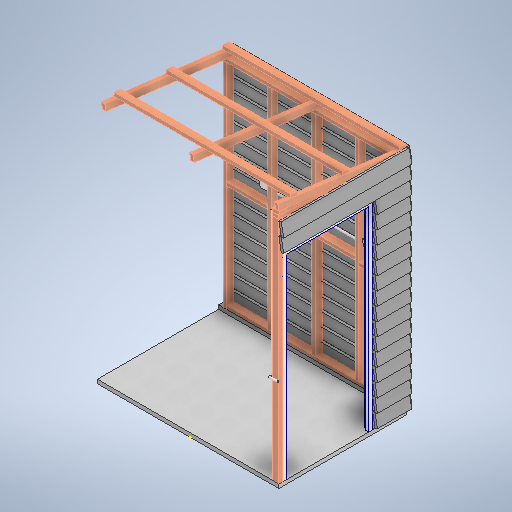
# Autodesk Inventor part: MaximaShed
Saved by Autodesk Inventor 2025 (Build 290162010, 162A)
## iProperties
Created: 2024-08-20
Part Number: MaximaShed
Material: Generic
Document SubType Name: Modeling
Designer: max_d
Density: 1 g/cm^3
Appearance: Default
Author: max_d
Autodesk Inventor part; units mm, degrees
ref_plane "YZ Plane" through (0, 0, 0) normal (1, 0, 0) x (0, 1, 0)
ref_plane "XZ Plane" through (0, 0, 0) normal (0, 1, 0) x (-1, 0, 0)
ref_plane "XY Plane" through (0, 0, 0) normal (0, 0, 1) x (1, 0, 0)
sketch "Sketch1" plane through (0, 0, 0) normal (0, 1, 0) x (-1, 0, 0)
  line L0 (0, 0) -> (-1850, 0)
  line L1 (-1850, 0) -> (-1850, -1235)
  line L2 (-1850, -1235) -> (0, -1235)
  line L3 (0, -1235) -> (0, 0)
  line L4 (0, -1235) -> (-1850, -1235)
  line L5 (-1850, -1235) -> (-1850, -1305)
  line L6 (-1850, -1305) -> (0, -1305)
  line L7 (0, -1305) -> (0, -1235)
  line L8 (-1850, -1235) -> (-1780, -1235)
  line L9 (-1780, -1235) -> (-1780, -975)
  line L10 (-1780, -975) -> (-1850, -975)
  line L11 (-1850, -975) -> (-1850, -1235)
  line L12 (-1780, -1105) -> (-1850, -1105) construction
  line L13 (-1744.6984, -1305) -> (-1744.6984, -1235) construction
  dimension "d0" = 1850
  dimension "d1" = 1235
  dimension "d5" = 70
  dimension "d19" = 260
  constraints: 28 end point, 6 parallel, 5 perpendicular, 3 horizontal, 2 midpoint, 2 point on line, 1 collinear
  measures "d0" distance of L2.end L1.end
  measures "d1" distance of L1.end L0.end
  measures "d5" distance of L5.end L4.end
  measures "d19" distance of L8.end L9.end
extrude "Extrusion1" add sketch "Sketch1" along normal blind 40 contours L3 L2 L9 L10 L1 L0 | L10 L9 L2 L1
extrude "Extrusion2" add sketch "Sketch1" along normal blind 80 contours L7 L6 L5 L2 | L10 L9 L2 L1
sketch "Sketch2" plane through (0, 80, 0) normal (0, 1, 0) x (1, 0, 0)
  line L0 (1850, 1305) -> (0, 1305) projected
  line L1 (0, 1235) -> (1780, 1235) projected
  line L2 (85, 1305) -> (85, 1235)
  line L3 (85, 1235) -> (50, 1235)
  line L4 (50, 1235) -> (50, 1305)
  line L5 (500, 1305) -> (535, 1305)
  line L6 (535, 1305) -> (535, 1235)
  line L7 (535, 1235) -> (500, 1235)
  line L8 (500, 1235) -> (500, 1305)
  line L9 (950, 1305) -> (985, 1305)
  line L10 (985, 1305) -> (985, 1235)
  line L11 (985, 1235) -> (950, 1235)
  line L12 (950, 1235) -> (950, 1305)
  line L13 (1395, 1305) -> (1430, 1305)
  line L14 (1430, 1305) -> (1430, 1235)
  line L15 (1430, 1235) -> (1395, 1235)
  line L16 (1395, 1235) -> (1395, 1305)
  line L17 (1850, 0) -> (1850, 1305) projected
  line L18 (1850, 1305) -> (1815, 1305)
  line L19 (1815, 1305) -> (1815, 1235)
  line L20 (1815, 1235) -> (1850, 1235)
  line L21 (1850, 1235) -> (1850, 1305)
  line L22 (1850, 1010) -> (1815, 1010)
  line L23 (1815, 1010) -> (1815, 975)
  line L24 (1815, 975) -> (1850, 975)
  line L25 (1850, 975) -> (1850, 1010)
  line L26 (1850, 0) -> (1815, 0)
  line L27 (1815, 0) -> (1815, 35)
  line L28 (1815, 35) -> (1850, 35)
  line L29 (1850, 35) -> (1850, 0)
  line L30 (50, 1270) -> (85, 1270) construction
  line L31 (85, 1270) -> (500, 1270) construction
  line L32 (500, 1270) -> (535, 1270) construction
  line L33 (535, 1270) -> (950, 1270) construction
  line L34 (950, 1270) -> (985, 1270) construction
  line L35 (985, 1270) -> (1395, 1270) construction
  line L36 (1395, 1270) -> (1430, 1270) construction
  line L37 (1430, 1270) -> (1815, 1270) construction
  line L38 (1832.5, 1235) -> (1832.5, 1010) construction
  line L39 (1832.5, 35) -> (1832.5, 0) construction
  line L40 (1832.5, 1010) -> (1832.5, 975) construction
  line L41 (1815, 1270) -> (1850, 1270) construction
  line L42 (0, 1305) -> (0, 1235) projected
  line L43 (50, 1305) -> (85, 1305)
  point P0 (0, 0)
  point P1 (500, 1305)
  point P2 (500, 1235)
  point P3 (535, 1305)
  point P4 (950, 1305)
  dimension "d8" = 35
  dimension "d9" = 385
  dimension "d10" = 225
  dimension "d88" = 410
  dimension "d89" = 415
  dimension "d90" = 50
  constraints: 80 end point, 15 midpoint, 13 parallel, 10 point on line, 6 equal length, 6 horizontal, 6 perpendicular, 1 collinear
  measures "d8" distance between parallel lines of L6 L8
  measures "d9" distance of L36.end L37.end
  measures "d10" distance of L38.start L38.end
  measures "d88" distance of L34.end L35.end
  measures "d89" distance of L32.end L33.end
  measures "d90" distance between parallel lines of L42 L4
extrude "Extrusion3" add sketch "Sketch2" along normal blind 2180 separate body contours L17 L20 L19 L0 | L14 L1 L16 L0 | L10 L1 L12 L0 | L6 L1 L8 L0 | L2 L1 L4 L0
sketch "Sketch3" plane through (85, 80, -1235) normal (1, 0, 0) x (0, 0, -1)
  line L0 (70, 0) -> (70, 2180) projected
  line L1 (0, 0) -> (70, 0)
  line L2 (70, 0) -> (70, 35)
  line L3 (70, 35) -> (0, 35)
  line L4 (0, 35) -> (0, 0)
  point P0 (-1235, -80)
  dimension "d13" = 35
  constraints: 8 end point, 2 parallel, 1 horizontal, 1 perpendicular, 1 point on line
  measures "d13" distance of L2.end L1.end
extrude "Extrusion4" cut sketch "Sketch3" along normal up to surface (1765 mm away) bodies 2
extrude "Extrusion5" add sketch "Sketch3" along normal up to surface (1765 mm away) separate body
sketch "Sketch4" plane through (85, 115, -1235) normal (0, 0, 1) x (1, 0, 0)
  line L0 (1765, 0) -> (1730, 0) projected
  line L1 (1695, -35) -> (1765, -35) projected
  line L2 (1765, 0) -> (1695, 0)
  line L3 (1695, 0) -> (1695, -35)
  line L4 (1695, -35) -> (1765, -35)
  line L5 (1765, -35) -> (1765, 0)
  point P0 (-85, -115)
  constraints: 8 end point, 2 parallel, 1 horizontal, 1 perpendicular
extrude "Extrusion6" add sketch "Sketch4" along normal up to surface (260 mm away) separate body
sketch "Sketch5" plane through (1780, 115, -1235) normal (0, 1, 0) x (1, 0, 0)
  line L0 (0, -260) -> (70, -260) projected
  line L1 (70, -1235) -> (70, 70) projected
  line L2 (0, -260) -> (70, -260)
  line L3 (70, -260) -> (70, -225)
  line L4 (70, -225) -> (0, -225)
  line L5 (0, -225) -> (0, -260)
  point P0 (-1780, -1235)
  dimension "d22" = 35
  constraints: 8 end point, 2 parallel, 1 horizontal, 1 perpendicular, 1 point on line
  measures "d22" distance between parallel lines of L0 L4
extrude "Extrusion7" add sketch "Sketch5" along normal blind 2170 separate body
sketch "Sketch6" plane through (1780, 115, -975) normal (0, 0, 1) x (1, 0, 0)
  point P0 (-1780, -115)
sketch "Sketch7" plane through (1780, 115, -975) normal (0, 0, 1) x (1, 0, 0)
  line L0 (0, 0) -> (0, 2170) projected
  line L1 (70, 0) -> (70, 2145) projected
  line L2 (0, 1990) -> (70, 1990)
  line L3 (70, 1990) -> (70, 1955)
  line L4 (70, 1955) -> (0, 1955)
  line L5 (0, 1955) -> (0, 1990)
  line L6 (-1780, -75) -> (70, -75) projected
  point P0 (-1780, -115)
  point P1 (0, 1955)
  point P2 (70, 1990)
  dimension "d25" = 35
  dimension "d26" = 2030
  constraints: 8 end point, 2 parallel, 2 point on line, 1 horizontal, 1 perpendicular
  measures "d25" distance between parallel lines of L4 L2
  measures "d26" distance between parallel lines of L6 L4
sketch "Sketch8" plane through (0, 40, 0) normal (0, 1, 0) x (1, 0, 0)
  line L0 (1850, 0) -> (1850, 1305) projected
  line L1 (1850, 0) -> (1780, 0)
  line L2 (1780, 0) -> (1780, 35)
  line L3 (1780, 35) -> (1850, 35)
  line L4 (1850, 35) -> (1850, 0)
  point P0 (0, 0)
  dimension "d27" = 70
  dimension "d28" = 35
  constraints: 8 end point, 2 parallel, 1 horizontal, 1 perpendicular
  measures "d27" distance of L2.end L3.end
  measures "d28" distance of L1.end L2.end
extrude "Extrusion8" add sketch "Sketch8" along normal blind 2335 separate body
extrude "Extrusion9" add sketch "Sketch7" along normal up to surface (940 mm away) separate body
sketch "Sketch9" plane through (1780, 2105, -975) normal (0, 1, 0) x (1, 0, 0)
  line L0 (70, -940) -> (3.3283, -940)
  line L1 (3.3283, -940) -> (3.3283, -905)
  line L2 (3.3283, -905) -> (70, -905)
  line L3 (70, -905) -> (70, -940)
  line L4 (0, 0) -> (0, -940) projected
  line L5 (70, -390) -> (0, -390)
  line L6 (0, -390) -> (0, -425)
  line L7 (0, -425) -> (70, -425)
  line L8 (70, -425) -> (70, -390)
  line L9 (70, 0) -> (0, 0) projected
  point P0 (-1780, -975)
  point P1 (0, -390)
  dimension "d33" = 35
  dimension "d34" = 35
  dimension "d35" = 390
  constraints: 16 end point, 4 parallel, 2 horizontal, 2 perpendicular, 2 point on line
  measures "d33" distance of L0.end L1.end
  measures "d34" distance of L6.end L5.end
  measures "d35" distance between parallel lines of L5 L9
extrude "Extrusion10" add sketch "Sketch9" along normal up to surface (270 mm away) separate body contours L0 L1 L2 L3
extrude "Extrusion11" add sketch "Sketch9" along normal blind 220 separate body contours L5 L8 L7 L4
sketch "Sketch10" plane through (50, 80, -1305) normal (-1, 0, 0) x (0, 0, 1)
  line L0 (70, 2180) -> (0, 2180) projected
  line L1 (0, 2180) -> (70, 2180)
  line L2 (70, 2180) -> (70, 2215)
  line L3 (70, 2215) -> (0, 2215)
  line L4 (0, 2215) -> (0, 2180)
  point P0 (1305, -80)
  dimension "d40" = 35
  constraints: 8 end point, 2 parallel, 1 horizontal, 1 perpendicular
  measures "d40" distance of L2.end L1.end
extrude "Extrusion12" add sketch "Sketch10" against normal up to surface (1800 mm away) separate body
sketch "Sketch11" plane through (1850, 2260, -1235) normal (1, 0, 0) x (0, 0, -1)
  line L0 (0, 0) -> (70, 0) projected
  line L1 (0, 0) -> (-1235, 115)
  line L2 (-503.8032, 82.0643) -> (-507.0483, 47.215) construction
  line L3 (-1235, -2220) -> (-1235, 115) construction
  line L4 (-1235, 115) -> (-1235, 150.1514)
  line L5 (-1235, 150.1514) -> (0, 35.1514)
  line L6 (0, 35.1514) -> (0, 0)
  point P0 (-1235, -2260)
  dimension "d45" = 35
  constraints: 10 end point, 2 perpendicular, 2 point on line, 2 vertical
  measures "d45" distance of L2.start L2.end
extrude "Extrusion13" cut sketch "Sketch11" against normal up to surface (70 mm away) bodies 5 9 8 6
extrude "Extrusion14" add sketch "Sketch11" against normal up to surface (70 mm away) separate body
sketch "Sketch12" plane through (1815, 2260, -1305) normal (-1, 0, 0) x (0, 0, 1)
  line L0 (0, -2145) -> (0, 0) projected
  line L1 (70, -2145) -> (70, 0) projected
  line L2 (0, -1090) -> (70, -1090)
  line L3 (70, -1090) -> (70, -1125)
  line L4 (70, -1125) -> (0, -1125)
  line L5 (0, -1125) -> (0, -1090)
  line L6 (0, -2145) -> (70, -2145) projected
  point P0 (1305, -2260)
  point P1 (0, -1125)
  point P2 (70, -1090)
  dimension "d50" = 35
  dimension "d51" = 1020
  constraints: 8 end point, 2 parallel, 2 point on line, 1 horizontal, 1 perpendicular
  measures "d50" distance of L2.end L3.end
  measures "d51" distance between parallel lines of L6 L4
extrude "Extrusion15" add sketch "Sketch12" along normal up to surface (385 mm away) separate body contours L0 L2 L1 L4
sketch "Sketch14" plane through (1850, 115, -1010) normal (0, 0, -1) x (-1, 0, 0)
  line L0 (0, 0) -> (0, 2165.9514) projected
  line L1 (70, 0) -> (70, 2165.9514) projected
  line L2 (0, 1055) -> (70, 1055)
  line L3 (70, 1055) -> (70, 1020)
  line L4 (70, 1020) -> (0, 1020)
  line L5 (0, 1020) -> (0, 1055)
  line L6 (35, 1055) -> (420, 1055) projected
  point P0 (1850, -115)
  point P1 (0, 1020)
  point P2 (70, 1055)
  dimension "d54" = 35
  constraints: 8 end point, 2 parallel, 2 point on line, 1 collinear, 1 horizontal, 1 perpendicular
  measures "d54" distance of L2.end L3.end
extrude "Extrusion16" add sketch "Sketch14" along normal up to surface (225 mm away) separate body
sketch "Sketch15" plane through (950, 2260, -1305) normal (-1, 0, 0) x (0, 0, 1)
  point P0 (1305, -2260)
sketch "Sketch16" plane through (950, 2260, -1305) normal (-1, 0, 0) x (0, 0, 1)
  line L0 (0, -2145) -> (0, 0) projected
  line L1 (70, -2145) -> (70, 0) projected
  line L2 (0, -1090) -> (70, -1090)
  line L3 (70, -1090) -> (70, -1125)
  line L4 (70, -1125) -> (0, -1125)
  line L5 (0, -1125) -> (0, -1090)
  line L6 (70, -1090) -> (0, -1090) projected
  point P0 (1305, -2260)
  point P1 (0, -1125)
  dimension "d57" = 35
  constraints: 8 end point, 2 parallel, 2 point on line, 1 collinear, 1 horizontal, 1 perpendicular
  measures "d57" distance of L2.end L3.end
sketch "Sketch17" plane through (1395, 2260, -1305) normal (-1, 0, 0) x (0, 0, 1)
  line L0 (0, -2145) -> (0, 0) projected
  line L1 (70, -2145) -> (70, 0) projected
  line L2 (0, -1055) -> (70, -1055)
  line L3 (70, -1055) -> (70, -1090)
  line L4 (70, -1090) -> (0, -1090)
  line L5 (0, -1090) -> (0, -1055)
  line L6 (70, -1090) -> (0, -1090) projected
  point P0 (1305, -2260)
  point P1 (70, -1055)
  dimension "d58" = 35
  constraints: 8 end point, 2 parallel, 2 point on line, 1 collinear, 1 horizontal, 1 perpendicular
  measures "d58" distance of L2.end L3.end
sketch "Sketch18" plane through (500, 2260, -1305) normal (-1, 0, 0) x (0, 0, 1)
  line L0 (0, -2145) -> (0, 0) projected
  line L1 (70, -2145) -> (70, 0) projected
  line L2 (0, -1090) -> (70, -1090)
  line L3 (70, -1090) -> (70, -1055)
  line L4 (70, -1055) -> (0, -1055)
  line L5 (0, -1055) -> (0, -1090)
  line L6 (70, -1090) -> (0, -1090) projected
  point P0 (1305, -2260)
  point P1 (0, -1055)
  dimension "d59" = 35
  constraints: 8 end point, 2 parallel, 2 point on line, 1 collinear, 1 horizontal, 1 perpendicular
  measures "d59" distance of L3.end L2.end
extrude "Extrusion17" add sketch "Sketch17" along normal up to surface (410 mm away) separate body
extrude "Extrusion18" add sketch "Sketch16" along normal up to surface (415 mm away) separate body
extrude "Extrusion19" add sketch "Sketch18" along normal up to surface (415 mm away) separate body
sketch "Sketch19" plane through (1850, 2260, -1235) normal (1, 0, 0) x (0, 0, -1)
  line L0 (0, 35.1514) -> (-1235, 150.1514) projected
  line L1 (-1235, 150.1514) -> (-1165.3015, 143.6613)
  line L2 (-1165.3015, 143.6613) -> (-1162.0564, 178.5105)
  line L3 (-1162.0564, 178.5105) -> (-1231.7549, 185.0007)
  line L4 (-1231.7549, 185.0007) -> (-1235, 150.1514)
  point P0 (-1235, -2260)
  dimension "d66" = 70
  dimension "d67" = 35
  constraints: 8 end point, 3 perpendicular, 1 point on line
  measures "d66" distance of L0.end L1.end
  measures "d67" distance of L1.end L2.end
extrude "Extrusion20" add sketch "Sketch19" against normal up to surface (70 mm away) separate body
sketch "Sketch20" plane through (1850, 2260, -1235) normal (1, 0, 0) x (0, 0, -1)
  line L0 (-1162.0564, 178.5105) -> (-1231.7549, 185.0007) projected
  line L1 (-1231.7549, 185.0007) -> (-1235, 150.1514) projected
  line L2 (0, 35) -> (70, 35) construction
  line L3 (-1162.0564, 178.5105) -> (0, 35)
  line L4 (0, 35.1514) -> (-1235, 150.1514) projected
  line L5 (0, 35.1514) -> (70, 35)
  line L6 (70, 35) -> (58.2612, 98.3367)
  line L7 (58.2612, 98.3367) -> (-1245.5351, 259.3517)
  line L8 (-1245.5351, 259.3517) -> (-1231.7549, 185.0007)
  line L9 (-1231.7549, 185.0007) -> (-1162.0564, 178.5105)
  line L10 (-896.0108, 145.6547) -> (-887.4312, 215.1269) construction
  line L11 (70, 35) -> (70, 0) projected
  point P0 (-1235, -2260)
  point P1 (-4.984, 35.6155)
  dimension "d72" = 70
  dimension "d144" = 10.5
  constraints: 14 end point, 3 parallel, 2 point on line, 1 perpendicular
  measures "d72" distance of L10.start L10.end
  measures "d144" angle of L11 L6
extrude "Extrusion21" add sketch "Sketch20" against normal blind 35 separate body contours L0 L8 L7 L6 L5 L4 L3
ref_plane "Work Plane1" through (950, 2260, -1235) normal (1, 0, 0) x (0, 0, -1)
mirror "Mirror1" about plane through (950, 2260, -1235) normal (1, 0, 0) of "Extrusion21" bodies 18
pattern_linear "Rectangular Pattern1" count 2 spacing 865 along (-1, 0, 0) of "Extrusion21" bodies 18
sketch "Sketch21" plane through (1850, 2260, -1235) normal (1, 0, 0) x (0, 0, -1)
  line L0 (-11.211, 106.9163) -> (-6.9212, 141.6524)
  line L1 (-6.9212, 141.6524) -> (62.551, 133.0728)
  line L2 (58.2612, 98.3367) -> (-1245.5351, 259.3517) projected
  line L3 (62.551, 133.0728) -> (58.2612, 98.3367)
  line L4 (58.2612, 98.3367) -> (-11.211, 106.9163)
  line L5 (-586.838, 178.0045) -> (-582.5482, 212.7406)
  line L6 (-582.5482, 212.7406) -> (-513.076, 204.161)
  line L7 (-513.076, 204.161) -> (-517.3658, 169.4249)
  line L8 (-517.3658, 169.4249) -> (-586.838, 178.0045)
  line L9 (-1117.8043, 243.5773) -> (-1113.5145, 278.3134)
  line L10 (-1113.5145, 278.3134) -> (-1044.0423, 269.7338)
  line L11 (-1044.0423, 269.7338) -> (-1048.3321, 234.9977)
  line L12 (-1048.3321, 234.9977) -> (-1117.8043, 243.5773)
  line L13 (-513.076, 204.161) -> (-6.9212, 141.6524) construction
  line L14 (-1044.0423, 269.7338) -> (-582.5482, 212.7406) construction
  point P0 (-1235, -2260)
  point P1 (-1117.8043, 243.5773)
  point P2 (-1048.3321, 234.9977)
  dimension "d78" = 35
  dimension "d79" = 70
  dimension "d80" = 35
  dimension "d81" = 70
  dimension "d82" = 35
  dimension "d83" = 70
  dimension "d84" = 510
  dimension "d85" = 465
  constraints: 28 end point, 7 perpendicular, 4 collinear, 1 point on line
  measures "d78" distance of L0.start L0.end
  measures "d79" distance of L0.end L1.end
  measures "d80" distance of L5.start L5.end
  measures "d81" distance of L5.end L6.end
  measures "d82" distance of L9.start L9.end
  measures "d83" distance of L9.end L10.end
  measures "d84" distance of L6.end L0.end
  measures "d85" distance of L5.end L10.end
extrude "Extrusion22" add sketch "Sketch21" against normal up to surface (1800 mm away) separate body
sketch "Sketch22" plane through (0, 40, 0) normal (0, 1, 0) x (1, 0, 0)
  line L0 (1850, 0) -> (1850, 975) projected
  line L1 (1850, 35) -> (1790, 35)
  line L2 (1790, 35) -> (1790, 55)
  line L3 (1790, 55) -> (1820, 55)
  line L4 (1820, 55) -> (1820, 75)
  line L5 (1820, 75) -> (1850, 75)
  line L6 (1850, 35) -> (1850, 75)
  line L7 (1850, 955) -> (1790, 955)
  line L8 (1790, 955) -> (1790, 935)
  line L9 (1790, 935) -> (1820, 935)
  line L10 (1820, 935) -> (1820, 915)
  line L11 (1820, 915) -> (1850, 915)
  line L12 (1850, 915) -> (1850, 955)
  line L13 (1850, 975) -> (1780, 975) projected
  line L14 (1850, 35) -> (1780, 35) projected
  point P0 (0, 0)
  dimension "d91" = 20
  dimension "d92" = 30
  dimension "d93" = 60
  dimension "d94" = 20
  dimension "d95" = 40
  dimension "d96" = 30
  dimension "d97" = 60
  dimension "d98" = 20
  dimension "d99" = 40
  constraints: 24 end point, 10 perpendicular, 4 point on line, 2 horizontal, 1 collinear
  measures "d91" distance between parallel lines of L7 L13
  measures "d92" distance of L10.end L11.end
  measures "d93" distance between parallel lines of L0 L8
  measures "d94" distance between parallel lines of L9 L7
  measures "d95" distance between parallel lines of L11 L7
  measures "d96" distance between parallel lines of L6 L4
  measures "d97" distance between parallel lines of L0 L2
  measures "d98" distance between parallel lines of L1 L3
  measures "d99" distance between parallel lines of L5 L1
extrude "Extrusion23" add sketch "Sketch22" along normal up to surface (2030 mm away) separate body
sketch "Sketch23" plane through (1850, 40, -955) normal (0, 0, -1) x (-1, 0, 0)
  line L0 (0, 2030) -> (0, 1990)
  line L1 (0, 0) -> (0, 2030) projected
  line L2 (0, 1990) -> (30, 1990)
  line L3 (30, 1990) -> (30, 2010)
  line L4 (30, 2010) -> (60, 2010)
  line L5 (60, 0) -> (60, 2030) projected
  line L6 (0, 2030) -> (60, 2030) projected
  line L7 (0, 2030) -> (60, 2030)
  line L8 (60, 2030) -> (60, 2010)
  point P0 (1850, -40)
  dimension "d102" = 40
  dimension "d103" = 20
  dimension "d104" = 30
  constraints: 12 end point, 4 perpendicular, 2 point on line, 1 collinear
  measures "d102" distance of L0.start L0.end
  measures "d103" distance of L2.end L3.end
  measures "d104" distance of L0.end L2.end
extrude "Extrusion24" add sketch "Sketch23" against normal up to surface (920 mm away) bodies 20
ref_plane "Work Plane2" through (0, 120, 0) normal (0, 1, 0) x (1, 0, 0)
sketch "Sketch25" plane through (0, 120, 0) normal (0, 1, 0) x (1, 0, 0)
  line L0 (0, 1305) -> (0, 0) projected
  line L1 (0, -55) -> (50, -55)
  line L2 (50, -55) -> (50, 15)
  line L3 (50, 15) -> (0, 15)
  line L4 (0, 15) -> (0, 0)
  line L5 (0, -55) -> (0, 15)
  line L6 (0, 0) -> (1850, 0) projected
  point P0 (0, 15)
  point P1 (50, 0)
  dimension "d112" = 50
  dimension "d113" = 70
  dimension "d122" = 15
  constraints: 10 end point, 2 collinear, 2 parallel, 1 horizontal, 1 perpendicular
  measures "d112" distance of L3.end L2.end
  measures "d113" distance of L2.end L1.end
  measures "d122" distance between parallel lines of L6 L3
extrude "Extrusion26" add sketch "Sketch25" along normal blind 2977.75 separate body
sketch "Sketch24" plane through (0, 80, -15) normal (0, 0, 1) x (1, 0, 0)
  line L0 (25.4179, 35.4478) -> (50, 40)
  line L1 (50, 40) -> (25.4179, 172.7431)
  line L2 (0, -40) -> (1850, -40) projected
  line L3 (25.4179, 35.4478) -> (0.8359, 168.1908)
  line L4 (0.8359, 168.1908) -> (25.4179, 172.7431)
  line L5 (50, 0) -> (50, 2180) projected
  line L6 (50, 40) -> (0, 40) projected
  point P0 (0, -80)
  dimension "d107" = 25
  dimension "d108" = 135
  constraints: 8 end point, 2 perpendicular, 1 parallel, 1 point on line, 1 vertical alignment, 2 other
  measures "d107" distance of L0.start L0.end
  measures "d108" distance of L0.end L1.end
extrude "Extrusion25" add sketch "Sketch24" against normal blind 1933.5 separate body
sketch "Sketch26" plane through (50, 120, 55) normal (1, 0, 0) x (0, 0, -1)
  line L0 (30.4179, -4.5522) -> (55, 0)
  line L1 (55, 0) -> (30.4179, 132.7431)
  line L2 (30.4179, -4.5522) -> (5.8359, 128.1908)
  line L3 (5.8359, 128.1908) -> (30.4179, 132.7431)
  line L4 (0, 0) -> (70, 0) projected
  line L5 (70, 0) -> (70, 2977.75) projected
  point P0 (55, -120)
  point P1 (29.5749, 0)
  dimension "d116" = 25
  dimension "d117" = 135
  dimension "d123" = 15
  constraints: 8 end point, 3 perpendicular, 1 point on line, 1 vertical alignment
  measures "d116" distance of L0.start L0.end
  measures "d117" distance of L0.end L1.end
  measures "d123" distance from line of L5 L0.end
extrude "Extrusion27" add sketch "Sketch26" along normal blind 2978.25 separate body
sketch "Sketch27" plane through (1850, 2260, -1235) normal (1, 0, 0) x (0, 0, -1)
  line L0 (94.5821, -2189.5522) -> (119.1641, -2185)
  line L1 (119.1641, -2185) -> (94.5821, -2052.2569)
  line L2 (94.5821, -2052.2569) -> (70, -2056.8092)
  line L3 (70, -2056.8092) -> (94.5821, -2189.5522)
  line L4 (70, -2145) -> (70, 0) projected
  line L5 (-1235, -2220) -> (-260, -2220) projected
  point P0 (-1235, -2260)
  dimension "d124" = 25
  dimension "d125" = 135
  dimension "d126" = 35
  constraints: 8 end point, 3 perpendicular, 1 point on line, 1 vertical alignment
  measures "d124" distance of L0.start L0.end
  measures "d125" distance of L0.end L1.end
  measures "d126" distance from line of L5 L0.end
extrude "Extrusion28" add sketch "Sketch27" against normal up to surface (1800 mm away) separate body
sketch "Sketch28" plane through (1815, 115, -1305) normal (0, 0, -1) x (-1, 0, 0)
  line L0 (-59.5821, -44.5522) -> (-84.1641, -40)
  line L1 (-84.1641, -40) -> (-59.5821, 92.7431)
  line L2 (-59.5821, 92.7431) -> (-35, 88.1908)
  line L3 (-35, 88.1908) -> (-59.5821, -44.5522)
  line L4 (-35, 0) -> (-35, 2145) projected
  line L5 (-35, -40) -> (1765, -40) projected
  point P0 (1815, -115)
  dimension "d129" = 25
  dimension "d130" = 135
  constraints: 8 end point, 3 perpendicular, 2 point on line, 1 vertical alignment
  measures "d129" distance of L0.start L0.end
  measures "d130" distance of L0.end L1.end
extrude "Extrusion29" add sketch "Sketch28" against normal up to surface (350 mm away) separate body
pattern_linear "Rectangular Pattern3" count 22 spacing 135 along (0, 1, 0) of "Extrusion27", "Extrusion25" bodies 23
pattern_linear "Rectangular Pattern4" count 17 spacing 135 along (0, 1, 0) of "Extrusion29", "Extrusion28" bodies 25
sketch "Sketch29" plane through (1874.5821, 70.4478, -955) normal (0, 0, 1) x (0.983282, 0.1820893, 0)
  line L0 (393.7308, 1991.1461) -> (369.1487, 1991.1461) projected
  line L1 (393.7308, 1991.1461) -> (368.7308, 1991.1461)
  line L2 (368.7308, 1993.403) -> (368.7308, 2126.1461) projected
  line L3 (368.7308, 1991.1461) -> (368.7308, 2126.1461)
  line L4 (368.7308, 2126.1461) -> (393.3128, 2126.1461)
  line L5 (393.3128, 2258.8891) -> (418.3128, 2258.8891) projected
  line L6 (393.3128, 2126.1461) -> (393.3128, 2258.8891)
  line L7 (393.3128, 2258.8891) -> (418.3128, 2258.8891)
  line L8 (418.3128, 2123.8891) -> (393.7308, 2123.8891) projected
  line L9 (418.3128, 2258.8891) -> (418.3128, 2123.8891)
  line L10 (418.3128, 2123.8891) -> (393.7308, 2123.8891)
  line L11 (393.7308, 2123.8891) -> (393.7308, 1991.1461)
  point P0 (-1856.0706, 272.0712)
  point P1 (368.7308, 1993.403)
  point P2 (369.1487, 1991.1461)
  constraints: 16 end point, 5 perpendicular, 2 collinear
extrude "Extrusion30" add sketch "Sketch29" along normal up to surface (955 mm away) bodies 25
sketch "Sketch30" plane through (50, 1287.667, -1329.1711) normal (0, -0.1820893, 0.983282) x (1, 0, 0)
  line L0 (450, -1135.9148) -> (450, 973.2251) projected
  line L1 (450, 0) -> (325, 0)
  line L2 (325, 0) -> (325, 80)
  line L3 (325, 80) -> (450, 80)
  line L4 (450, 80) -> (450, 0)
  line L5 (1800, 0) -> (0, 0) projected
  line L6 (1380, -1148.661) -> (1380, 960.4789) projected
  line L7 (1380, 0) -> (1505, 0)
  line L8 (1505, 0) -> (1505, 80)
  line L9 (1505, 80) -> (1380, 80)
  line L10 (1380, 80) -> (1380, 0)
  point P0 (-50, -1024.112)
  point P1 (1380, 80)
  dimension "d145" = 125
  dimension "d146" = 80
  constraints: 16 end point, 4 parallel, 2 collinear, 2 equal length, 2 horizontal, 2 perpendicular, 2 point on line
  measures "d145" distance of L2.end L3.end
  measures "d146" distance between parallel lines of L1 L3
extrude "Extrusion31" add sketch "Sketch30" along normal blind 45 separate body
sketch "Sketch31" plane through (375, 1287.667, -1329.1711) normal (-1, 0, 0) x (0, -0.1820893, 0.983282)
  circle A0 centre (25, 10) radius 10
  line L0 (0, 0) -> (45, 0) projected
  line L1 (0, 80) -> (0, 0) projected
  point P0 (1541.4203, -1024.112)
  dimension "d149" = 20
  dimension "d167" = 25
  constraints: 1 centre point, 1 tangent
  measures "d149" diameter of A0
  measures "d167" distance from line of L1 A0.centre
sketch3d "3D Sketch1"
  line L0 (375, 1292.9476, -1302.7681) -> (1805, 1292.9476, -1302.7681)
  line L1 (1805, 1292.9476, -1302.7681) -> (1805, 2250, -1302.7681)
  line L2 (1805, 2250, -1302.7681) -> (1805, 2250, -1225)
  line L3 (1805, 2250, -1225) -> (1770, 2250, -1225)
  line L4 (1770, 2250, -1225) -> (1770, 2305, -1225)
  line L5 (1770, 2305, -1225) -> (1805, 2305, -1225)
  line L6 (1805, 2305, -1225) -> (1805, 2412.7453, -80)
  line L7 (1805, 2412.7453, -80) -> (1770, 2412.7453, -80)
  line L8 (1770, 2412.7453, -80) -> (1770, 2412.7453, -10)
  line L9 (1770, 2412.7453, -10) -> (1770, 950, -10)
  line L10 (1770, 950, -10) -> (1770, 950, 10)
  line L11 (1770, 950, 10) -> (1850, 950, 10)
  dimension "d151" = 10
  dimension "d152" = 10
  dimension "d153" = 10
  dimension "d154" = 10
  dimension "d155" = 10
  dimension "d157" = 10
  dimension "d158" = 10
  dimension "d159" = 10
  dimension "d160" = 10
  dimension "d161" = -10
  dimension "d162" = 910
  dimension "d163" = 10
  dimension "d164" = 0
sweep "Sweep1" add profiles "Sketch31" path "3D Sketch1" bodies 26
sketch "Sketch32" plane through (0, 0, 0) normal (1, 0, 0) x (0, 1, 0)
  line L0 (2225, -290) -> (1210, -290)
  line L1 (1210, -290) -> (1210, -1060)
  line L2 (1210, -1060) -> (2225, -1060)
  line L3 (2225, -1060) -> (2225, -290)
  line L4 (40, -1235) -> (40, 0) projected
  line L5 (80, -1305) -> (2260, -1305) projected
  point P0 (0, 0)
  dimension "d168" = 770
  dimension "d169" = 1015
  dimension "d170" = 1170
  dimension "d172" = 245
  constraints: 8 end point, 2 parallel, 1 horizontal, 1 perpendicular
  measures "d168" distance of L0.end L1.end
  measures "d169" distance of L1.end L2.end
  measures "d170" distance between parallel lines of L4 L1
  measures "d172" distance between parallel lines of L2 L5
extrude "Extrusion32" cut sketch "Sketch32" along normal mid plane 779.25 bodies 23
body "Solid1"
body "Solid2"
body "Solid3"
body "Solid4"
body "Solid5"
body "Solid6"
body "Solid7"
body "Solid8"
body "Solid9"
body "Solid10"
body "Solid11"
body "Solid12"
body "Solid13"
body "Solid14"
body "Solid15"
body "Solid16"
body "Solid17"
body "Solid18"
body "Solid19"
body "Solid20"
body "Solid22"
body "Solid23"
body "Solid24"
body "Solid25"
body "Solid26"
body "Solid28"
